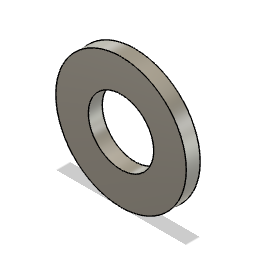
Epi-EndoAssembly (Autodesk Fusion 360 archive; units mm, degrees)
design "Plain Washer ANSI B18.22.1 - #8 - Narrow - Type B Steel 100 HV Plain"
description: Plain Washer ANSI B18.22.1 - #8 - Narrow - Type B
Autodesk Fusion 360 part; units mm, degrees
sketch "Sketch1" plane through (0, 0, 0) normal (0, 0, 1) x (1, 0, 0)
  circle A0 centre (0, 0) radius 4.7625
  circle A1 centre (0, 0) radius 2.3876
  dimension "d4" = 9.525
  dimension "d5" = 4.7752
  constraint coincident A0.centre A1.centre
  measures "d4" diameter of A0
  measures "d5" diameter of A1
extrude "Extrude2" add sketch "Sketch1" along normal blind 1.016
equation "d4 = adsk_woutdia"
equation "d5 = adsk_windia"
equation "adsk_woutdia = 0.375 in"
equation "adsk_windia = 0.188 in"
equation "adsk_wthick = 0.04 in"
equation "d20 = adsk_wthick"
equation "d41 = adsk_wthick"

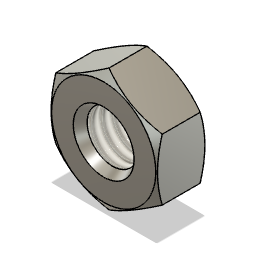
design "Hexagon Regular Nut ISO 4032 - M4 Steel 6 Plain"
description: Hexagon Regular Nut ISO 4032 - M4
Autodesk Fusion 360 part; units mm, degrees
sketch "Sketch1" plane through (0, 0, 0) normal (0, 1, 0) x (1, 0, 0)
  line L0 (0, 0) -> (0, -3.2)
  line L1 (-2, 0) -> (-3.43, 0)
  line L2 (-3.43, 0) -> (-4.0425, -0.3536)
  line L3 (-4.0425, -0.3536) -> (-4.0425, -2.8464)
  line L4 (-4.0425, -2.8464) -> (-3.43, -3.2)
  line L5 (-3.43, -3.2) -> (-2, -3.2)
  line L6 (-2, -3.2) -> (-2, 0)
  dimension "d121" = 4
  dimension "d122" = 30
  dimension "d123" = 30
  dimension "d126" = 3.2
  dimension "d128" = 8.085
  dimension "d172" = 6.86
  constraint vertical L0
  constraint coincident L0 L0.end
  constraint coincident origin L0
  constraint horizontal L1
  constraint perpendicular L1 L3
  constraint perpendicular L3 L5
  constraint perpendicular L5 L6
  constraint coincident L0.start L1
  constraint coincident L0.start origin
  constraint coincident L0.end L5
  constraint equal L1 L5
  measures "d122" angle of L1 L2
  measures "d123" angle of L4 L5
  measures "d126" distance of L1.start L5.end
revolve "Revolve1" add sketch "Sketch1" angle 360 about axis through (0, 0, 0) along (0, 0, 1)
sketch "Sketch8" plane through (0, 0, 3.2) normal (0, 0, 1) x (1, 0, 0)
  line L0 (0, 0) -> (-7, 0) construction
  line L1 (-3.5, -2.0228) -> (-3.5, 2.0228)
  circle A0 centre (0, 0) radius 2
  circle A1 centre (0, 0) radius 4.0425
  dimension "d114" = 3.5
  constraint horizontal L0
  constraint perpendicular L0 L1
  constraint midpoint L0 L1
  constraint coincident L0.start A0.centre
  constraint coincident L1.end A1
  measures "d114" distance of L0.start L1
extrude "Extrude5" cut sketch "Sketch8" against normal blind 3.2 contours L1 A1 picked at (-3.5875, -0.4927)
pattern_circular "C-Pattern2" count 6 over 360 about axis through (0, 0, 1.75) along (0, 0, 1) of "Extrude5"
thread "Thread3" "ISO Metric profile 4.0 M4x0.7 6H" major diameter 4.1095 minor diameter 3.332 pitch 0.7 angle 60 resizes the face on face at (-1.9975, 0.0997, 2.1333)
sketch "Sketch12" plane through (0, 0, 0) normal (0, 1, 0) x (1, 0, 0)
  line L0 (1.666, -3.2) -> (-1.666, -3.2)
  line L1 (3.43, -3.2) -> (-3.43, -3.2)
  line L2 (3.43, 0) -> (-3.43, 0)
  line L3 (1.666, 0) -> (-1.666, 0)
  line L4 (-2, 0) -> (0, 0)
  line L5 (-1.0762, -1.6) -> (-2, 0)
  line L6 (-2, -3.2) -> (0, -3.2)
  line L7 (-1.0762, -1.6) -> (-2, -3.2)
  line L8 (0, 0) -> (0, -3.2)
  dimension "d165" = 60
  dimension "d169" = 60
  dimension "d170" = 2
  constraint horizontal L4
  constraint collinear L1 L6
  constraint coincident L5.start L7.start
  constraint vertical L4.start L6.start
  constraint coincident L1 L6.end
  constraint coincident L6.end L8.end
  constraint coincident L4.end L8.start
  measures "d165" angle of L2 L5
  measures "d169" angle of L6 L7
  measures "d170" distance of L4.start L4.end
revolve "Revolve3" cut sketch "Sketch12" angle 360 about axis through (0, 0, 1.75) along (0, 0, 1)
equation "adsk_nheig = 3.20 mm"
equation "adsk_maxdia = 8.085 mm"
equation "adsk_nomdia = 4.00 mm"
equation "d89 = -adsk_nheig"
equation "adsk_waflat = 7.00 mm"
equation "d114 = adsk_waflat / 2"
equation "adsk_chamang1 = 30.00 deg"
equation "adsk_chamang2 = 30.00 deg"
equation "d121 = adsk_nomdia"
equation "d122 = adsk_chamang1"
equation "d123 = adsk_chamang2"
equation "d126 = adsk_nheig"
equation "d128 = adsk_maxdia"
equation "d163 = adsk_nheig"
equation "d170 = adsk_nomdia * 0.5"
equation "adsk_beardia = adsk_waflat * 0.98"
equation "d172 = adsk_beardia"

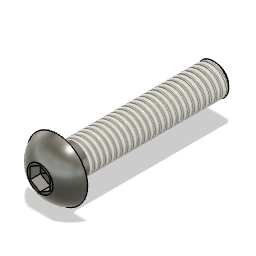
design "Hexagon Socket Button Head Screw ISO 7380-1 - M4 x 20 Steel 4.6 Plain"
description: Hexagon Socket Button Head Screw ISO 7380-1 - M4 x 20
Autodesk Fusion 360 part; units mm, degrees
sketch "Sketch1" plane through (0, 0, 0) normal (0, 1, 0) x (1, 0, 0)
  line L0 (-2, 0) -> (-2, 20)
  line L1 (-2, 20) -> (0, 20)
  line L2 (0, 20) -> (0, -2.2)
  line L3 (-2, 0) -> (-3.8, 0)
  line L4 (0, -2.2) -> (-1.625, -2.2)
  arc A0 (-3.8, 0) -> (-1.625, -2.2) centre (0, 1.5817) ccw
  dimension "d9" = 4
  dimension "d66" = 7.6
  dimension "d68" = 20
  dimension "d98" = 3.25
  dimension "d99" = 2.2
  constraint perpendicular L0 L1
  constraint perpendicular L0 L3
  constraint coincident origin L3
  constraint vertical L0
  constraint vertical L2
  constraint coincident origin L2
  constraint perpendicular L2 L4
  constraint coincident L2 A0.centre
  measures "d68" distance of origin L1.end
  measures "d99" vertical distance of L2.end L3.end
revolve "Revolve1" add sketch "Sketch1" angle 360 about axis through (0, 0, -20) along (0, 0, 1)
ref_plane "WorkPlane1" through (0, 0, 2.2) normal (0, 0, 1) x (1, 0, 0)
sketch "Sketch6" plane through (0, 0, 2.2) normal (0, 0, 1) x (1, 0, 0)
  line L0 (-1.25, 0) -> (1.25, 0) construction
  line L1 (0, 0) -> (-1.25, 0.7217)
  line L2 (-1.25, -0.7217) -> (-1.25, 0.7217)
  line L3 (-1.25, -0.7217) -> (0, 0)
  dimension "d72" = 2.5
  dimension "d91" = 150
  constraint horizontal L0
  constraint midpoint L1.start L0
  constraint coincident L1.start L3.end
  constraint perpendicular L0 L2
  constraint midpoint L0.start L2
  constraint coincident L1.end L2.end
  measures "d72" distance of L0.start L0.end
  measures "d91" angle of L0 L1
extrude "Extrude1" cut sketch "Sketch6" against normal blind 1.3
pattern_circular "C-Pattern1" count 6 over 360 about axis through (0, 0, 1.75) along (0, 0, 1) of "Extrude1"
extrude "Extrude2" cut 1 faces at (-0.4167, -0.2406, 0.9) along direction (0, 0, -1) blind 1.3 draft -85
fillet "Fillet5" radius 0.4 1 edges at (-1.8647, 0.7232, 0)
thread "Thread2" "ISO Metric profile 4.0 M4x0.7 6g" major diameter 3.908 minor diameter 3.111 pitch 0.7 angle 60 resizes the face on face at (-1.9901, 0.1991, -6.9333) from (0, 0, -2.1) to (0, 0, -20)
sketch "Sketch5" plane through (0, 0, 0) normal (0, 1, 0) x (1, 0, 0)
  line L0 (0, 20) -> (0, -2.2)
  line L1 (0, 20) -> (-2.04, 20)
  line L2 (-2.04, 20) -> (-2.04, 19.5706)
  line L3 (-2.04, 19.5706) -> (-1.5706, 20)
  dimension "d92" = 1.5706
  dimension "d93" = 2.04
  dimension "d94" = 0.4294
  constraint coincident L0.start L1.start
  constraint perpendicular L0 L1
  constraint perpendicular L1 L2
  constraint coincident L1 L3.end
  measures "d92" horizontal distance of origin L3.end
  measures "d93" horizontal distance of origin L1.end
  measures "d94" distance of L1.end L2.end
revolve "Revolve2" cut sketch "Sketch5" angle 360 about axis through (0, 0, -20) along (0, 0, 1)
equation "d9 = adsk_nomdia"
equation "adsk_nomlen = 20.00 mm"
equation "adsk_headh = 2.20 mm"
equation "adsk_headdia = 7.60 mm"
equation "adsk_nomdia = 4.00 mm"
equation "adsk_philwidth = 2.50 mm"
equation "d31 = -adsk_phildepth"
equation "adsk_phildepth = 1.30 mm"
equation "d66 = adsk_headdia"
equation "d68 = adsk_nomlen"
equation "d71 = adsk_headh"
equation "d72 = adsk_philwidth"
equation "d76 = -adsk_phildepth"
equation "adsk_thrlen = 17.90 mm"
equation "adsk_endpointdia = adsk_nomdia - 2 * adsk_startlen"
equation "adsk_startlen = 0.429415 mm"
equation "d92 = adsk_endpointdia / 2"
equation "d93 = adsk_nomdia * 0.51"
equation "d94 = adsk_startlen"
equation "d96 = adsk_thrlen"
equation "d98 = adsk_philwidth * 1.3"
equation "d99 = adsk_headh"
equation "adsk_midfillet = 0.40 mm"
equation "d104 = adsk_midfillet"
